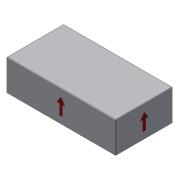
# Autodesk Inventor part: Bloco de NdFeB - N45SH.
Saved by Autodesk Inventor 2016 (Build 200138000, 138)
## iProperties
Created: 2014-09-22
Part Number: Bloco de NdFeB - N45SH.
Material: NdFeB (Neodímio Ferro Boro)
Document SubType Name: Modeling
Designer: reinaldo.basilio
Density: 7.6 g/cm^3
Description: Bloco magnético de NdFeB cód. N45SH.
Mass: 1316.7 g
Surface Area: 211.5 cm^2
Volume: 173.25 cm^3
Appearance: White
Project: DIPOLO 2 T - BC- SIRIUS.
Cost Center: 1504002005
Author: reinaldo.basilio
Title: DIPOLO 2 T - BC- SIRIUS.
Subject: Bloco de NdFeB - N45SH.
Autodesk Inventor part; units mm, degrees
ref_plane "YZ Plane" through (0, 0, 0) normal (1, 0, 0) x (0, 1, 0)
ref_plane "XZ Plane" through (0, 0, 0) normal (0, 1, 0) x (-1, 0, 0)
ref_plane "XY Plane" through (0, 0, 0) normal (0, 0, 1) x (1, 0, 0)
sketch "Sketch1" plane through (0, 0, 0) normal (0, 0, 1) x (1, 0, 0)
  line L0 (0, 38.5) -> (0, -38.5) projected
  line L1 (-73.5, 0) -> (73.5, 0) projected
  line L2 (-52.5, 27.5) -> (52.5, 27.5)
  line L3 (52.5, 27.5) -> (52.5, -27.5)
  line L4 (52.5, -27.5) -> (-52.5, -27.5)
  line L5 (-52.5, -27.5) -> (-52.5, 27.5)
  point P0 (0, 0)
  point P1 (0, 27.5)
  point P2 (52.5, 0)
  dimension "d0" = 55
  dimension "d1" = 105
  constraints: 8 end point, 2 midpoint, 2 parallel, 2 point on line, 1 horizontal, 1 perpendicular
  measures "d0" distance of L4.end L2.start
  measures "d1" distance of L2.start L2.end
extrude "Extrusion1" add sketch "Sketch1" along normal blind 30
chamfer "Chamfer1" distance 0.5 angle 45 12 edges at (0, -27.5, 30) (-52.5, 0, 30) (0, 27.5, 30) (52.5, 0, 30) (52.5, 27.5, 15) (52.5, -27.5, 15) (-52.5, -27.5, 15) (0, -27.5, 0) (52.5, 0, 0) (0, 27.5, 0) (-52.5, 27.5, 15) (-52.5, 0, 0)
sketch "Sketch2" plane through (-52, -27.5, 0.5) normal (0, -1, 0) x (1, 0, 0)
  line L0 (0, 0) -> (0, 29) projected
  line L1 (52, 22.5) -> (48, 16.5)
  line L2 (48, 16.5) -> (56, 16.5)
  line L3 (56, 16.5) -> (52, 22.5)
  line L4 (50.5, 16.5) -> (53.5, 16.5)
  line L5 (53.5, 16.5) -> (53.5, 6.5)
  line L6 (53.5, 6.5) -> (50.5, 6.5)
  line L7 (50.5, 6.5) -> (50.5, 16.5)
  line L8 (52, 22.5) -> (52, 4.7859)
  line L9 (104, 29.5) -> (0, 29.5) projected
  point P0 (52, -0.5)
  dimension "d7" = 8
  dimension "d8" = 3
  dimension "d9" = 4
  dimension "d10" = 1.5
  dimension "d11" = 7
  dimension "d12" = 6
  dimension "d13" = 10
  constraints: 16 end point, 2 parallel, 2 perpendicular, 1 horizontal, 1 point on line, 1 vertical
  measures "d7" distance of L1.end L2.end
  measures "d8" distance of L5.end L6.end
  measures "d9" distance from line of L8 L2.end
  measures "d10" distance between parallel lines of L8 L5
  measures "d11" distance from line of L9 L1.start
  measures "d12" vertical distance of L2.end L1.start
  measures "d13" distance between parallel lines of L2 L6
extrude "Extrusion2" cut sketch "Sketch2" against normal blind 0.025
sketch "Sketch3" plane through (-52, 27.5, 0.5) normal (0, 1, 0) x (1, 0, 0)
  line L0 (53.5, -6.5) -> (50.5, -6.5)
  line L1 (52, -22.5) -> (48, -16.5)
  line L2 (48, -16.5) -> (56, -16.5)
  line L3 (56, -16.5) -> (52, -22.5)
  line L4 (53.5, -16.5) -> (53.5, -6.5)
  line L5 (50.5, -6.5) -> (50.5, -16.5)
  line L6 (0, -29.5) -> (104, -29.5) projected
  line L7 (50.5, -6.5) -> (53.5, -6.5)
  line L8 (53.5, -6.5) -> (53.5, -16.5)
  line L9 (50.5, -16.5) -> (53.5, -16.5)
  line L10 (50.5, -16.5) -> (50.5, -6.5)
  point P0 (52, 0.5)
  point P1 (52, -6.5)
  dimension "d17" = 3
  dimension "d25" = 7
  constraints: 20 end point, 2 collinear, 2 perpendicular, 1 midpoint, 1 point on line
  measures "d17" distance of L0.start L0.end
  measures "d25" distance from line of L6 L1.start
extrude "Extrusion3" cut sketch "Sketch3" against normal blind 0.025
sketch "Sketch4" plane through (52.5, -27, 0.5) normal (1, 0, 0) x (0, 0, -1)
  line L0 (-22.5, 27) -> (-16.5, 23)
  line L1 (-16.5, 23) -> (-16.5, 31)
  line L2 (-16.5, 31) -> (-22.5, 27)
  line L3 (-16.5, 25.5) -> (-16.5, 28.5)
  line L4 (-16.5, 28.5) -> (-6.5, 28.5)
  line L5 (-6.5, 28.5) -> (-6.5, 25.5)
  line L6 (-6.5, 25.5) -> (-16.5, 25.5)
  line L7 (-22.5, 27) -> (-5.1122, 27)
  line L8 (-29.5, 54) -> (-29.5, 0) projected
  point P0 (0.5, 27)
  dimension "d37" = 74.49
  dimension "d39" = 3
  dimension "d40" = 8
  dimension "d41" = 16
  dimension "d42" = 6
  dimension "d43" = 1.5
  dimension "d44" = 67.38
  dimension "d45" = 7
  dimension "d48" = 7
  constraints: 16 end point, 2 vertical, 1 horizontal, 1 horizontal alignment, 1 point on line
  measures "d39" distance between parallel lines of L6 L4
  measures "d40" distance of L0.end L1.end
  measures "d41" distance from line of L0.start L5
  measures "d42" distance from line of L0.start L1
  measures "d43" distance between parallel lines of L7 L4
  measures "d44" angle of L0 L2
  measures "d45" distance from line of point (0.5, 27) L5
  measures "d48" distance from line of L8 L0.start
extrude "Extrusion4" cut sketch "Sketch4" against normal blind 0.025
sketch "Sketch5" plane through (-52.5, -27, 0.5) normal (-1, 0, 0) x (0, 0, 1)
  line L0 (22.5, 27) -> (16.5, 23)
  line L1 (16.5, 23) -> (16.5, 31)
  line L2 (16.5, 31) -> (22.5, 27)
  line L3 (16.5, 25.5) -> (16.5, 28.5)
  line L4 (16.5, 28.5) -> (6.5, 28.5)
  line L5 (6.5, 28.5) -> (6.5, 25.5)
  line L6 (6.5, 25.5) -> (16.5, 25.5)
  line L7 (22.5, 27) -> (5.6122, 27)
  line L8 (29.5, 0) -> (29.5, 54) projected
  point P0 (-0.5, 27)
  point P1 (29.5, 27)
  dimension "d57" = 16
  dimension "d58" = 7
  dimension "d59" = 3
  dimension "d60" = 1.5
  dimension "d61" = 67.38
  dimension "d62" = 6
  constraints: 16 end point, 2 point on line, 1 horizontal, 1 horizontal alignment, 1 midpoint
  measures "d57" horizontal distance of L7.start L5.start
  measures "d58" distance from line of L8 L7.start
  measures "d59" distance between parallel lines of L6 L4
  measures "d60" distance between parallel lines of L4 L7
  measures "d61" angle of L0 L2
  measures "d62" distance from line of L7.start L1
extrude "Extrusion5" cut sketch "Sketch5" against normal blind 0.025
equation "\"d9\" = 0.5 * d7"
equation "\"d10\" = 0.5 * d8"
body "Solid1"
